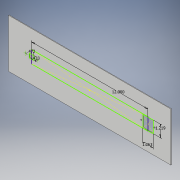
# Autodesk Inventor part: back
Saved by Autodesk Inventor 2017 (Build 210142000, 142)
## iProperties
Created: 2016-09-21
Part Number: back
Material: Generic
Document SubType Name: Modeling
Designer: Darien Morrow
Density: 1 g/cm^3
Appearance: Default
Author: Darien Morrow
Autodesk Inventor part; units mm, degrees
ref_plane "YZ Plane" through (0, 0, 0) normal (1, 0, 0) x (0, 1, 0)
ref_plane "XZ Plane" through (0, 0, 0) normal (0, 1, 0) x (-1, 0, 0)
ref_plane "XY Plane" through (0, 0, 0) normal (0, 0, 1) x (1, 0, 0)
sketch "Sketch1" plane through (0, 0, 0) normal (0, 0, 1) x (1, 0, 0)
  line L0 (-212.725, -63.5) -> (212.725, -63.5)
  line L1 (212.725, -63.5) -> (212.725, 63.5)
  line L2 (212.725, 63.5) -> (-212.725, 63.5)
  line L3 (-212.725, 63.5) -> (-212.725, -63.5)
  line L4 (-212.725, -63.5) -> (212.725, 63.5) construction
  line L5 (212.725, -63.5) -> (-212.725, 63.5) construction
  point P0 (0, 0)
  dimension "d0" = 127
  dimension "d1" = 425.45
  constraints: 12 end point, 2 midpoint, 2 parallel, 1 horizontal, 1 perpendicular
  measures "d0" distance between parallel lines of L0 L2
  measures "d1" distance between parallel lines of L1 L3
extrude "Extrusion1" add sketch "Sketch1" along normal blind 1.5875
sketch "Sketch2" plane through (0, 0, 1.5875) normal (0, 0, 1) x (1, 0, 0)
  line L0 (152.4, -16.2954) -> (-152.4, -16.2954)
  line L1 (-152.4, -16.2954) -> (-152.4, 16.2954)
  line L2 (-152.4, 16.2954) -> (152.4, 16.2954)
  line L3 (152.4, 16.2954) -> (152.4, -16.2954)
  line L4 (152.4, -16.2954) -> (-152.4, 16.2954) construction
  line L5 (-152.4, -16.2954) -> (152.4, 16.2954) construction
  line L6 (-158.4, -5.4991) -> (-146.4, -5.4991)
  line L7 (-146.4, -5.4991) -> (-146.4, 5.4991)
  line L8 (-146.4, 5.4991) -> (-158.4, 5.4991)
  line L9 (-158.4, 5.4991) -> (-158.4, -5.4991)
  line L10 (-158.4, -5.4991) -> (-146.4, 5.4991) construction
  line L11 (-146.4, -5.4991) -> (-158.4, 5.4991) construction
  line L12 (138.9062, -15.4813) -> (165.8937, -15.4813)
  line L13 (165.8937, -15.4813) -> (165.8937, 15.4813)
  line L14 (165.8937, 15.4813) -> (138.9062, 15.4813)
  line L15 (138.9062, 15.4813) -> (138.9062, -15.4813)
  line L16 (138.9062, -15.4813) -> (165.8937, 15.4813) construction
  line L17 (165.8937, -15.4813) -> (138.9062, 15.4813) construction
  point P0 (0, 0)
  point P1 (-137.8966, 0)
  point P2 (-166.9034, 0)
  dimension "d4" = 304.8
  dimension "d5" = 12
  dimension "d6" = 10.9982
  dimension "d9" = 26.9875
  dimension "d10" = 30.9626
  constraints: 36 end point, 6 parallel, 3 horizontal, 3 perpendicular, 2 midpoint
  measures "d4" distance between parallel lines of L3 L1
  measures "d5" distance between parallel lines of L7 L9
  measures "d6" distance between parallel lines of L6 L8
  measures "d9" distance between parallel lines of L13 L15
  measures "d10" distance between parallel lines of L12 L14
extrude "Extrusion2" cut sketch "Sketch2" against normal up to next contours L12 L15 L14 L3 | L3 L14 L13 L12 | L6 L9 L8 L1 | L1 L8 L7 L6
sketch "Sketch3" plane through (0, 0, 1.5875) normal (0, 0, 1) x (1, 0, 0)
  point P0 (0, 0)
hole "Hole1" at (-166.9034, 0, 1.5875) at (-137.8966, 0, 1.5875) direction (0, 0, -1) diameter 3.4036 end through all clearance for "Flat Head Machine Screw" size "M3" standard "Ansi Metric M Profile"
sketch "Sketch4" plane through (0, 0, 1.5875) normal (0, 0, 1) x (1, 0, 0)
  point P0 (0, 0)
  point P1 (169.8625, 0)
  point P2 (134.9375, 0)
  point P3 (152.4, 0)
  dimension "d22" = 34.925
  dimension "d23" = 17.4625
  dimension "d24" = 152.4
  measures "d22" distance of point (134.938, 0) point (169.863, 0)
  measures "d23" distance of point (134.938, 0) point (152.4, 0)
  measures "d24" distance of point (152.4, 0) point (0, 0)
hole "Hole2" at (134.9375, 0, 1.5875) at (169.8625, 0, 1.5875) direction (0, 0, -1) diameter 3.2766 end through all clearance for "Flat Head Machine Screw (82)" size "#4" standard "Ansi Unified Screw Threads"
body "Solid1"
